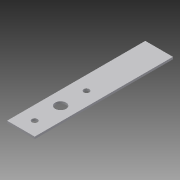
# Autodesk Inventor part: X Bar
Saved by Autodesk Inventor 2013 (Build 170138000, 138)
## iProperties
Created: 2013-01-27
Part Number: X Bar
Material: Generic
Document SubType Name: Modeling
Designer: carneeki
Density: 1 g/cm^3
Author: carneeki
Autodesk Inventor part; units mm, degrees
ref_plane "YZ Plane" through (0, 0, 0) normal (1, 0, 0) x (0, 1, 0)
ref_plane "XZ Plane" through (0, 0, 0) normal (0, 1, 0) x (-1, 0, 0)
ref_plane "XY Plane" through (0, 0, 0) normal (0, 0, 1) x (1, 0, 0)
sketch "Sketch1" plane through (0, 0, 0) normal (0, 0, 1) x (1, 0, 0)
  line L0 (-12.7, 1) -> (12.7, 1)
  line L1 (12.7, 1) -> (12.7, -1)
  line L2 (12.7, -1) -> (-12.7, -1)
  line L3 (-12.7, -1) -> (-12.7, 1)
  point P0 (0, 0)
  dimension "d0" = 25.4
  dimension "d1" = 2
  dimension "d2" = 12.7
  dimension "d3" = 1
  constraints: 8 end point, 2 parallel, 1 horizontal, 1 perpendicular
  measures "d0" distance between parallel lines of L1 L3
  measures "d1" distance between parallel lines of L0 L2
  measures "d2" distance from line of point (0, 0) L1
  measures "d3" distance from line of point (0, 0) L0
extrude "Extrusion1" add sketch "Sketch1" against normal blind 177.8
sketch "Sketch2" plane through (-12.7, 1, 0) normal (0, 1, 0) x (1, 0, 0)
  line L0 (25.4, 0) -> (25.4, 177.8) projected
  circle A0 centre (12.7, 12.7) radius 2.5908
  circle A1 centre (12.7, 138.1125) radius 2.5908
  circle A2 centre (12.7, 60.325) radius 2.5908
  line L1 (0, 0) -> (25.4, 0) projected
  line L2 (0, 0) -> (0, 177.8) projected
  line L3 (12.7, 60.325) -> (12.7, 12.7) construction
  line L4 (0, 36.5125) -> (25.4, 36.5125) construction
  point P0 (12.7, 0)
  dimension "d6" = 5.1816
  dimension "d7" = 12.7
  dimension "d8" = 12.7
  dimension "d9" = 5.1816
  dimension "d18" = 5.1816
  dimension "d19" = 47.625
  dimension "d26" = 36.5125
  dimension "d27" = 101.6
  constraints: 4 end point, 3 centre point, 2 point on line, 1 parallel, 1 perpendicular, 1 vertical alignment
  measures "d6" diameter of A0
  measures "d7" distance from line of L0 L3.end
  measures "d8" distance of point (12.7, 0) L3.end
  measures "d9" diameter of A1
  measures "d18" diameter of A2
  measures "d19" distance of L3.end L3.start
  measures "d26" distance between parallel lines of L1 L4
  measures "d27" distance from line of L4 A1.centre
hole "Hole1" at (0, 1, -138.1125) at (0, 1, -12.7) at (0, 1, -60.325) direction (0, -1, 0) diameter 5.1816 end through all
sketch "Sketch3" plane through (-12.7, 1, 0) normal (0, 1, 0) x (1, 0, 0)
  circle A0 centre (12.7, 36.5125) radius 5
  circle A1 centre (12.7, 12.7) radius 2.5908 projected
  circle A2 centre (12.7, 60.325) radius 2.5908 projected
  line L0 (0, 0) -> (25.4, 0) projected
  line L1 (25.4, 0) -> (25.4, 177.8) projected
  line L2 (0, 0) -> (0, 177.8) projected
  line L3 (12.7, 60.325) -> (12.7, 12.7) construction
  line L4 (0, 36.5125) -> (25.4, 36.5125) construction
  point P0 (12.7, 0)
  point P1 (12.7, 36.5125)
  point P2 (12.7, 36.5125)
  dimension "d20" = 10
  dimension "d24" = 36.5125
  constraints: 4 end point, 2 coincident, 2 midpoint, 2 point on line, 1 centre point, 1 parallel, 1 perpendicular
  measures "d20" diameter of A0
  measures "d24" distance between parallel lines of L0 L4
extrude "Extrusion2" cut sketch "Sketch3" against normal through all contours A0
equation "\"d2\" = 0.5 * d0"
equation "\"d3\" = 0.5 * d1"
equation "\"d8\" = d7"
body "Solid1"
